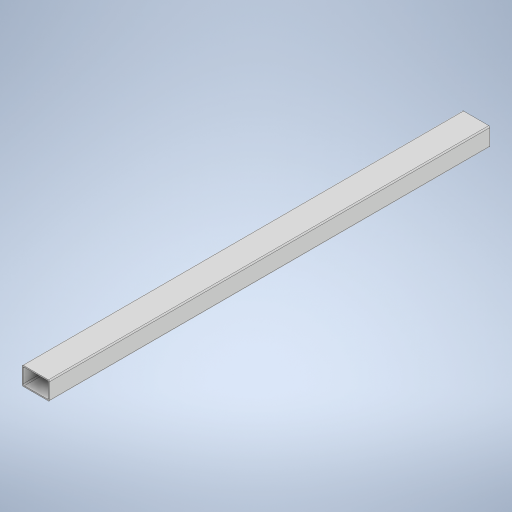
# Autodesk Inventor part: 2x3_Tube
Saved by Autodesk Inventor 2023 (Build 270158000, 158)
## iProperties
Created: 2022-05-03
Part Number: 2x3_Tube
Material: Generic
Document SubType Name: Modeling
Designer: plebbb
Density: 1 g/cm^3
Appearance: Default
Mass: 934.063 g
Surface Area: 5766.27 cm^2
Volume: 934.063 cm^3
Author: plebbb
Autodesk Inventor part; units mm, degrees
ref_plane "YZ Plane" through (0, 0, 0) normal (1, 0, 0) x (0, 1, 0)
ref_plane "XZ Plane" through (0, 0, 0) normal (0, 1, 0) x (-1, 0, 0)
ref_plane "XY Plane" through (0, 0, 0) normal (0, 0, 1) x (1, 0, 0)
sketch "Sketch1" plane through (0, 0, 0) normal (0, 0, 1) x (1, 0, 0)
  line L0 (0, 0) -> (76.2, 0)
  line L1 (76.2, 0) -> (76.2, 50.8)
  line L2 (76.2, 50.8) -> (0, 50.8)
  line L3 (0, 50.8) -> (0, 0)
  dimension "d0" = 76.2
  dimension "d1" = 50.8
  constraints: 8 end point, 2 parallel, 1 horizontal, 1 perpendicular
  measures "d0" distance of L1.end L2.end
  measures "d1" distance of L0.end L1.end
extrude "Extrusion1" add sketch "Sketch1" along normal blind 1219.2
shell "Shell1" thickness 3.175 removed faces 2 at (50.8, 16.9333, 1219.2) at (50.8, 16.9333, 0)
fillet "Fillet1" radius 3.175 8 edges at (0, 50.8, 609.6) (3.175, 47.625, 609.6) (76.2, 50.8, 609.6) (73.025, 47.625, 609.6) (3.175, 3.175, 609.6) (0, 0, 609.6) (76.2, 0, 609.6) (73.025, 3.175, 609.6)
body "Solid1"
